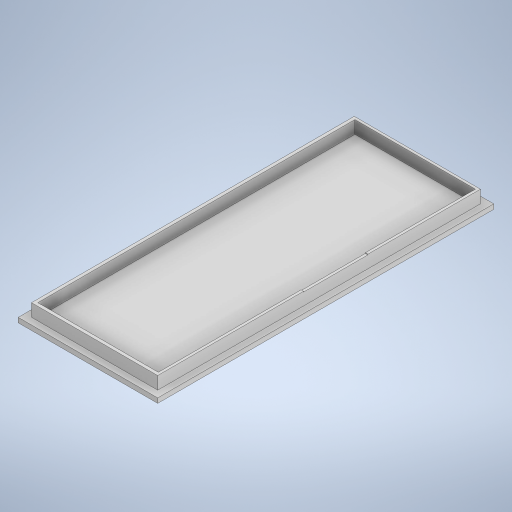
# Autodesk Inventor part: roller_deck_01_10_2025
Saved by Autodesk Inventor 2024.2 (Build 282272000, 272)
## iProperties
Created: 2025-08-30
Part Number: roller_deck_01_10_2025
Material: Типовые
Document SubType Name: Modeling
Designer: winds
Density: 1 g/cm^3
Appearance: По умолчанию
Author: winds
Autodesk Inventor part; units mm, degrees
ref_plane "YZ Plane" through (0, 0, 0) normal (1, 0, 0) x (0, 1, 0)
ref_plane "XZ Plane" through (0, 0, 0) normal (0, 1, 0) x (-1, 0, 0)
ref_plane "XY Plane" through (0, 0, 0) normal (0, 0, 1) x (1, 0, 0)
sketch "плоскость" plane through (0, 0, 0) normal (0, 1, 0) x (-1, 0, 0)
  line L0 (0, 0) -> (44, 0)
  line L1 (44, 0) -> (44, -106)
  line L2 (44, -106) -> (0, -106)
  line L3 (0, -106) -> (0, 0)
  dimension "d0" = 106
  dimension "d1" = 44
  constraints: 8 end point, 2 parallel, 1 horizontal, 1 perpendicular
  measures "d0" distance of L0.end L1.end
  measures "d1" distance of L0.start L0.end
extrude "Выдавливание1" add sketch "плоскость" along normal blind 1.5
sketch "Эскиз2" plane through (0, 1.5, 0) normal (0, 1, 0) x (1, 0, 0)
  line L0 (-41.9, 2.1) -> (-2.1, 2.1)
  line L1 (-2.1, 2.1) -> (-2.1, 103.9)
  line L2 (-2.1, 103.9) -> (-41.9, 103.9)
  line L3 (-41.9, 103.9) -> (-41.9, 2.1)
  line L4 (-44, 0) -> (0, 0) projected
  line L5 (-44, 106) -> (-44, 0) projected
  dimension "d4" = 39.8
  dimension "d5" = 101.8
  dimension "d6" = 2.1
  dimension "d20" = 2.1
  constraints: 8 end point, 2 parallel, 1 horizontal, 1 perpendicular
  measures "d4" distance of L0.start L0.end
  measures "d5" distance between parallel lines of L2 L0
  measures "d6" distance between parallel lines of L0 L4
  measures "d20" distance between parallel lines of L5 L3
extrude "Выдавливание2" add sketch "Эскиз2" along normal blind 4
sketch "Эскиз3" plane through (0, 5.5, 0) normal (0, 1, 0) x (1, 0, 0)
  line L0 (-40.9, 3.1) -> (-2.9, 3.1)
  line L1 (-2.9, 3.1) -> (-2.9, 103.1)
  line L2 (-2.9, 103.1) -> (-40.9, 103.1)
  line L3 (-40.9, 103.1) -> (-40.9, 3.1)
  line L4 (-41.9, 103.9) -> (-41.9, 2.1) projected
  line L5 (-41.9, 2.1) -> (-2.1, 2.1) projected
  point P0 (0, 0)
  dimension "d10" = 38
  dimension "d11" = 100
  dimension "d12" = 1
  dimension "d13" = 1
  constraints: 8 end point, 2 parallel, 1 horizontal, 1 perpendicular
  measures "d10" distance of L0.start L0.end
  measures "d11" distance of L2.end L0.start
  measures "d12" distance between parallel lines of L4 L3
  measures "d13" distance between parallel lines of L5 L0
extrude "Выдавливание3" cut sketch "Эскиз3" against normal blind 4
sketch "Эскиз7" plane through (-2.1, 1.5, -2.1) normal (1, 0, 0) x (0, 0, -1)
  line L0 (101, 4) -> (1, 4) projected
  line L1 (66.3, 3.8) -> (46, 3.8)
  line L2 (46, 3.8) -> (46, 4)
  line L3 (46, 4) -> (66.3, 4)
  line L4 (66.3, 4) -> (66.3, 3.8)
  line L5 (101.8, 0) -> (101.8, 4) projected
  point P0 (-2.1, -1.5)
  point P1 (66.3, 4)
  point P2 (101.8, 2)
  point P3 (66.3, 3.9)
  point P4 (51, 4)
  dimension "d18" = 35.5
  dimension "d19" = 0.2
  constraints: 8 end point, 3 midpoint, 2 parallel, 1 horizontal, 1 perpendicular, 1 point on line
  measures "d18" horizontal distance of point (101.8, 2) point (66.3, 3.9)
  measures "d19" distance from line of point (51, 4) L1
extrude "Выдавливание4" cut sketch "Эскиз7" against normal blind 2
